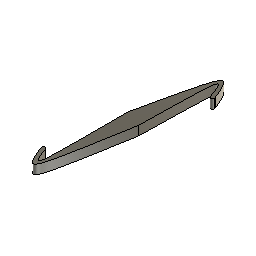
hang (Autodesk Fusion 360 design; units mm, degrees)
Autodesk Fusion 360 part; units mm, degrees
sketch "Sketch1" plane through (0, 0, 0) normal (0, 0, 1) x (1, 0, 0) in component "Component"
  spline S0 degree 2 poles (10, 80) (5.0297, 93.4362) (4.2042, 46.769) knots 0 0 0 4.658728 4.658728 4.658728 weights 1 3 1
  spline S1 degree 2 poles (12.0706, 80) (5.1934, 97.2023) (-5, 50) knots 0 0 0 5.205587 5.205587 5.205587 weights 1 3 1
  circle A0 centre (11.0353, 80) radius 1.0353
  circle A1 centre (-10.8941, 10) radius 1.0353
  spline S2 degree 2 poles (-11.9294, 10) (-5.0522, -7.2023) (4.2042, 46.769) knots 0 0 0 5.693161 5.693161 5.693161 weights 1 3 1
  spline S3 degree 2 poles (-9.8588, 10) (-4.8885, -3.4362) (-5, 50) knots 0 0 0 5.175631 5.175631 5.175631 weights 1 3 1
  constraint coincident S1.start A0
  constraint coincident S0.start A0
  constraint coincident S2.start A1
  constraint coincident S3.start A1
extrude "Extrude1" add sketch "Sketch1" along normal blind 5 contours S1 A0 | S0 S1 A0 A1 S2 S3 | A1 S2 picked at (10.7842, 79.7746) picked at (-11.1089, 9.7783) in component "Component"
component "Component" placed x (1, 0, 0) y (0, 1, 0) z (0, 0, 1) at (0, 0, 0)
